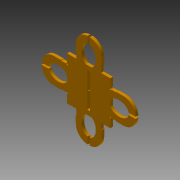
# Autodesk Inventor part: Lock2
Saved by Autodesk Inventor 2014 SP2 (Build 180246200, 246)
## iProperties
Created: 2014-11-24
Part Number: Lock2
Material: Generic
Document SubType Name: Modeling
Designer: JLM
Density: 1 g/cm^3
Appearance: Default
Author: JLM
Autodesk Inventor part; units mm, degrees
ref_plane "YZ Plane" through (0, 0, 0) normal (1, 0, 0) x (0, 1, 0)
ref_plane "XZ Plane" through (0, 0, 0) normal (0, 1, 0) x (-1, 0, 0)
ref_plane "XY Plane" through (0, 0, 0) normal (0, 0, 1) x (1, 0, 0)
sketch "Sketch1" plane through (0, 0, 0) normal (0, 0, 1) x (1, 0, 0)
  line L0 (48.35, 0) -> (48.35, 13.2)
  line L1 (48.35, 13.2) -> (28.35, 13.2)
  line L2 (28.35, 13.2) -> (28.35, 12.7)
  line L3 (28.35, 12.7) -> (22.25, 12.7)
  line L4 (12.2521, 0) -> (48.35, 0)
  line L5 (22.25, 12.7) -> (22.25, 22.25)
  line L6 (22.25, 22.25) -> (0, 22.25)
  line L7 (48.35, 1) -> (41.2217, 1)
  line L8 (48.35, 0) -> (48.35, -13.2)
  line L9 (48.35, -13.2) -> (28.35, -13.2)
  line L10 (28.35, -13.2) -> (28.35, -12.7)
  line L11 (28.35, -12.7) -> (22.25, -12.7)
  line L12 (22.25, -12.7) -> (22.25, -22.25)
  line L13 (22.25, -22.25) -> (0, -22.25)
  line L14 (48.35, -1) -> (41.2217, -1)
  line L15 (0, 22.25) -> (0, -22.25)
  ellipse E0 centre (31.324, 0) end of major axis (41.3133, 0) minor radius 7.4028 (41.2217, 1) -> (41.2217, -1) ccw
  point P0 (0, 0)
  point P1 (17.8114, 0)
  point P2 (41.275, 1)
  point P3 (41.275, -1)
  dimension "d0" = 13.2
  dimension "d1" = 20
  dimension "d6" = 12.7
  dimension "d7" = 22.25
  dimension "d8" = 22.25
  dimension "d9" = 6.1
  dimension "d17" = 48.35
  dimension "d29" = 6.1
  dimension "d31" = 1
  dimension "d32" = 44.5
  constraints: 32 end point, 8 symmetric about line, 7 point on line, 4 perpendicular, 2 parallel, 4 other
  measures "d0" distance of L0.start L0.end
  measures "d1" distance of L0.end L1.end
  measures "d6" distance between parallel lines of L4 L3
  measures "d7" distance between parallel lines of L4 L6
  measures "d8" distance from line of L5 point (0, 0)
  measures "d9" distance of L2.end L3.end
  measures "d17" distance from line of L8 point (0, 0)
  measures "d29" distance of L11.start L12.start
  measures "d31" distance between parallel lines of L4 L7
  measures "d32" distance between parallel lines of L13 L6
extrude "Extrusion2" add sketch "Sketch1" along normal blind 2.794 contours L7 E0 L14 L8 L9 L10 L11 L12 L13 L15 L6 L5 L3 L2 L1 L0
pattern_circular "Circular Pattern1" count 4 over 360 about axis through (0, 0, -10) along (0, 0, 1) of "Extrusion2"
fillet "Fillet2" radius 12.7 2 edges at (48.35, 13.2, 1.397) (48.35, -13.2, 1.397)
fillet "Fillet3" radius 12.7 6 edges at (-48.35, -13.2, 1.397) (-48.35, 13.2, 1.397) (-13.2, 48.35, 1.397) (13.2, 48.35, 1.397) (-13.2, -48.35, 1.397) (13.2, -48.35, 1.397)
sketch "Sketch2" plane through (0, 0, 2.794) normal (0, 0, 1) x (1, 0, 0)
  line L0 (-1.5, -17.5) -> (1.5, -17.5)
  line L1 (1.5, -17.5) -> (1.5, 17.5)
  line L2 (1.5, 17.5) -> (-1.5, 17.5)
  line L3 (-1.5, 17.5) -> (-1.5, -17.5)
  line L4 (-1.5, -17.5) -> (1.5, 17.5) construction
  line L5 (1.5, -17.5) -> (-1.5, 17.5) construction
  point P0 (0, 0)
  dimension "d23" = 3
  dimension "d24" = 35
  constraints: 12 end point, 2 midpoint, 2 parallel, 1 horizontal, 1 perpendicular
  measures "d23" distance of L2.end L1.end
  measures "d24" distance of L1.end L0.end
extrude "Extrusion3" cut sketch "Sketch2" against normal up to next
hole "Hole1" at (22.2343, 12.688, 2.794) direction (0, 0, -1) diameter 2 end through all
mirror "Mirror1" about plane through (0, 0, 0) normal (0, 1, 0) of "Hole1"
mirror "Mirror2" about plane through (0, 0, 0) normal (1, 0, 0) of "Hole1", "Mirror1"
equation "\"d7\" = d8"
body "Solid2"
